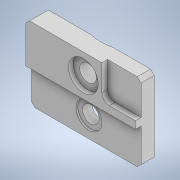
# Autodesk Inventor part: rd-mount
Saved by Autodesk Inventor 2020 (Build 240168000, 168)
## iProperties
Created: 2021-02-05
Part Number: rd-mount
Material: Generic
Document SubType Name: Modeling
Designer: maria
Density: 1 g/cm^3
Appearance: Default
Mass: 2.33213 g
Surface Area: 17.3346 cm^2
Volume: 2.33213 cm^3
ItemSpecifications: {"_id":"604686e30f193700099c8e30","finish":"543ef1f380da5b0c476373c1","finish_location":null,"material":"5515e170db035c20ce34af9a","process_initialism":null,"quotes":null,"current_quote":null,"quantity_ordered":1,"features":null,"hardware":null,"threading":null,"part_markings":[],"surface_roughness":null,"tolerance":null,"weld_quantity":null,"Notes":"","certifications":[],"part":null,"revision_num":0,"last_history":null,"inspection_requirement_details":{"inspection_requirement":"std","customer_data_sheet":null},"feedback":null}
ItemSpecifications: {"_id":"601dc59aa32ada0009083b59","finish":"543ef1f380da5b0c476373c1","finish_location":null,"material":"5515e170db035c20ce34af9a","process_initialism":null,"quotes":null,"current_quote":null,"quantity_ordered":1,"features":null,"hardware":null,"threading":null,"part_markings":[],"surface_roughness":null,"tolerance":null,"weld_quantity":null,"Notes":"","certifications":[],"part":null,"revision_num":0,"last_history":null,"inspection_requirement_details":{"inspection_requirement":"std","customer_data_sheet":null},"feedback":null}
Author: maria
Autodesk Inventor part; units mm, degrees
ref_plane "YZ Plane" through (0, 0, 0) normal (1, 0, 0) x (0, 1, 0)
ref_plane "XZ Plane" through (0, 0, 0) normal (0, 1, 0) x (-1, 0, 0)
ref_plane "XY Plane" through (0, 0, 0) normal (0, 0, 1) x (1, 0, 0)
sketch "Sketch1" plane through (0, 0, 0) normal (0, 0, 1) x (1, 0, 0)
  line L0 (-15.5, 11) -> (14, 11)
  line L1 (14, 11) -> (14, -10)
  line L2 (14, -10) -> (-15.5, -10)
  line L3 (-15.5, -10) -> (-15.5, 11)
  point P0 (0, 0)
  dimension "d0" = 29.5
  dimension "d1" = 21
  dimension "d2" = 10
  dimension "d3" = 14
  constraints: 8 end point, 2 parallel, 1 horizontal, 1 perpendicular
  measures "d0" distance of L0.start L0.end
  measures "d1" distance of L0.end L1.end
  measures "d2" distance from line of L2 point (0, 0)
  measures "d3" distance from line of L1 point (0, 0)
extrude "Extrusion1" add sketch "Sketch1" against normal blind 3.55
sketch "Sketch2" plane through (0, 0, 0) normal (0, 0, 1) x (1, 0, 0)
  line L0 (-15.5, 11) -> (14, 11)
  line L1 (14, 11) -> (14, 0)
  line L2 (14, 0) -> (-15.5, 0)
  line L3 (-15.5, 0) -> (-15.5, 11)
  line L4 (14, 11) -> (-15.5, 11) projected
  point P0 (0, 0)
  dimension "d6" = 29.5
  dimension "d8" = 0
  dimension "d27" = 0
  dimension "d77" = 14
  constraints: 8 end point, 2 parallel, 1 horizontal, 1 perpendicular
  measures "d6" distance of L0.start L0.end
  measures "d8" distance from line of point (0, 0) L2
  measures "d27" distance between parallel lines of L4 L0
  measures "d77" distance from line of L1 point (0, 0)
extrude "Extrusion2" add sketch "Sketch2" along normal blind 1.5
sketch "Sketch3" plane through (0, 0, 1.5) normal (0, 0, 1) x (1, 0, 0)
  line L0 (-15.5, 0) -> (14, 0) projected
  line L1 (14, 11) -> (-15.5, 11) projected
  point P0 (0, 0)
  point P1 (0, 5.5)
  dimension "d12" = 0
  dimension "d28" = 11
  dimension "d29" = 5.5
  measures "d12" horizontal distance of point (0, 0) point (0, 5.5)
  measures "d28" distance between parallel lines of L0 L1
  measures "d29" distance of point (0, 5.5) point (0, 0)
sketch "Sketch5" plane through (0, 0, -3.55) normal (0, 0, -1) x (-1, 0, 0)
  line L0 (15.5, -10) -> (15.5, 11) projected
  line L1 (-14, 0) -> (15.5, 0) projected
  line L2 (-14, -10) -> (15.5, -10) projected
  line L3 (-14, -10) -> (-14, 0) projected
  point P0 (0, 0)
  point P1 (0, -4.5)
  dimension "d19" = 4.5
  dimension "d78" = 14
  measures "d19" distance of point (0, 0) point (0, -4.5)
  measures "d78" distance from line of L3 point (0, -4.5)
hole "Hole1" at (0, -4.5, -3.55) direction (0, 0, 1) diameter 4.5 end through all counterbore diameter 7.94 counterbore depth 0.5 clearance for "Socket Head Cap Screw" size "#8" standard "Ansi Unified Screw Threads"
hole "Hole2" at (0, 5.5, 1.5) direction (0, 0, -1) diameter 4.5 end through all counterbore diameter 8 counterbore depth 1.25 clearance for "Socket Head Cap Screw" size "#8" standard "Ansi Unified Screw Threads"
sketch "Sketch6" plane through (0, 0, -3.55) normal (0, 0, -1) x (-1, 0, 0)
  line L0 (5.498, 5.5) -> (4.502, 5.5) construction
  line L1 (5.498, 6.55) -> (4.502, 6.55)
  line L2 (4.502, 4.45) -> (5.498, 4.45)
  arc A0 (5.498, 4.45) -> (5.498, 6.55) centre (5.498, 5.5) ccw
  arc A1 (4.502, 6.55) -> (4.502, 4.45) centre (4.502, 5.5) ccw
  point P0 (0, 0)
  point P1 (0, 5.5)
  point P2 (-5, 5.5)
  point P3 (5, 5.5)
  dimension "d37" = 0
  dimension "d38" = 5.5
  dimension "d39" = 0
  dimension "d40" = 5
  dimension "d41" = 0
  dimension "d42" = 5
  dimension "d58" = 1.05
  dimension "d60" = 0.996
  constraints: 8 end point, 4 point on circle, 4 tangent, 2 centre point, 1 horizontal, 1 midpoint, 1 parallel
  measures "d37" horizontal distance of point (0, 0) point (0, 5.5)
  measures "d38" distance of point (0, 5.5) point (0, 0)
  measures "d39" vertical distance of point (0, 5.5) point (5, 5.5)
  measures "d40" distance of point (0, 5.5) point (5, 5.5)
  measures "d41" vertical distance of point (0, 5.5) point (-5, 5.5)
  measures "d42" distance of point (0, 5.5) point (-5, 5.5)
  measures "d58" radius of A1
  measures "d60" distance of L0.start L0.end
hole "Hole3" at (5, 5.5, -3.55) direction (0, 0, 1) diameter 2.1 depth 2
sketch "Sketch8" plane through (0, 0, 0) normal (0, 0, 1) x (1, 0, 0)
  circle A0 centre (0, -4.5) radius 3.5
  circle A1 centre (0, -4.5) radius 2.25 projected
  point P0 (0, 0)
  dimension "d53" = 0
  dimension "d54" = 0
  dimension "d55" = 7
  constraints: 1 centre point
  measures "d53" distance of A1.centre A0.centre
  measures "d54" distance of A1.centre A0.centre
  measures "d55" diameter of A0
extrude "Extrusion3" cut sketch "Sketch8" against normal blind 0.5
extrude "Extrusion4" cut sketch "Sketch6" against normal blind 2.1
chamfer "Chamfer3" distance 1 angle 45 4 edges at (14, 11, -1.025) (-15.5, 11, -1.025) (14, -10, -1.775) (-15.5, -10, -1.775)
sketch "Sketch9" plane through (-14.5, 11, 1.5) normal (0, 1, 0) x (1, 0, 0)
  circle A0 centre (14.5, 17.4) radius 12.7
  line L0 (27.5, 0) -> (0, 0) projected
  point P0 (14.5, 1.5)
  point P1 (30, 0)
  point P2 (0.5, 0)
  dimension "d72" = 0
  dimension "d73" = 25.4
  dimension "d74" = 17.4
  constraints: 1 centre point
  measures "d72" horizontal distance of point (14.5, 1.5) A0.centre
  measures "d73" diameter of A0
  measures "d74" distance from line of A0.centre L0
extrude "Extrusion5" cut sketch "Sketch9" against normal up to surface (21 mm away)
sketch "Sketch10" plane through (-14.5, 11, 1.5) normal (0, 1, 0) x (1, 0, 0)
  circle A0 centre (23.017, -3.75) radius 5.25
  line L0 (27.5, 0) -> (0, 0) projected
  point P0 (14.5, 1.5)
  point P1 (19.3428, 0)
  point P2 (26.6912, 0)
  dimension "d79" = 10.5
  dimension "d82" = 3.75
  dimension "d83" = 8.517
  constraints: 1 centre point
  measures "d79" diameter of A0
  measures "d82" distance from line of L0 A0.centre
  measures "d83" horizontal distance of point (14.5, 1.5) A0.centre
extrude "Extrusion6" [suppressed]
sketch "Sketch11" plane through (0, 0, 1.5) normal (0, 0, 1) x (1, 0, 0)
  line L0 (5, 11) -> (14, 11)
  line L1 (14, 11) -> (14, 2)
  line L2 (14, 2) -> (7, 2)
  line L3 (5, 4) -> (5, 11)
  line L4 (13, 11) -> (-14.5, 11) projected
  line L5 (14, 0) -> (14, 10) projected
  line L6 (-15.5, 0) -> (14, 0) projected
  arc A0 (5, 4) -> (7, 2) centre (7, 4) ccw
  point P0 (0, 0)
  point P1 (5, 2)
  point P2 (4.8428, 11)
  point P3 (12.1912, 0)
  dimension "d86" = 0
  dimension "d87" = 0
  dimension "d88" = 9
  dimension "d89" = 2
  dimension "d94" = 2
  constraints: 8 end point, 2 parallel, 2 point on circle, 2 point on line, 2 tangent, 1 centre point, 1 horizontal, 1 perpendicular
  measures "d86" distance between parallel lines of L4 L0
  measures "d87" distance between parallel lines of L5 L1
  measures "d88" distance of L0.start L0.end
  measures "d89" distance between parallel lines of L6 L2
  measures "d94" radius of A0
extrude "Extrusion7" cut sketch "Sketch11" against normal blind 1.5
equation "\"d6\" = d0"
equation "\"d77\" = d3"
equation "\"d29\" = 0.5 * d28"
equation "\"d78\" = d3"
equation "\"d40\" = d42"
body "Solid1"
